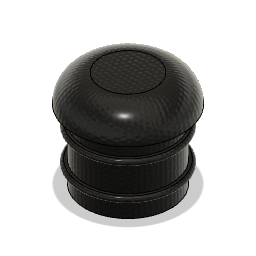
tube_cap (Autodesk Fusion 360 design; units mm, degrees)
Autodesk Fusion 360 part; units mm, degrees
sketch "Esquisse1" plane through (0, 0, 0) normal (0, 1, 0) x (1, 0, 0)
  circle A0 centre (0, 0) radius 8
  circle A1 centre (0, 0) radius 6
  dimension "d1" = 16
  dimension "d2" = 12
  constraint coincident A0.centre A1.centre
  measures "d1" diameter of A0
  measures "d2" diameter of A1
extrude "Extrusion1" add sketch "Esquisse1" along normal blind 10
sketch "Esquisse2" plane through (0, 10, 0) normal (0, 1, 0) x (-1, 0, 0)
  circle A0 centre (0, 0) radius 6
  circle A1 centre (0, 0) radius 8
  circle A2 centre (0, 0) radius 10
  dimension "d5" = 20
  constraint concentric A0 A2
  measures "d5" diameter of A2
extrude "Extrusion2" add sketch "Esquisse2" along normal blind 5 contours A0 | A1 | A2
fillet "Congé1" radius 5 1 edges at (9.3233, 15, -3.6162)
move_face "DécalerLesFaces1" offset -7 1 faces at (7.3035, 0, 0.3974)
sketch "Esquisse3" plane through (0, 7, 0) normal (0, -1, 0) x (1, 0, 0)
  circle A0 centre (0, 0) radius 6
  circle A1 centre (0, 0) radius 8
  circle A2 centre (0, 0) radius 6
  circle A3 centre (0, 0) radius 9
  dimension "d11" = 18
  constraint concentric A0 A2
  constraint coincident A0.centre A1.centre
  measures "d11" diameter of A3
extrude "Extrusion3" add sketch "Esquisse3" along normal blind 1 contours A1 | A3
sketch "Esquisse4" plane through (0, 6, 0) normal (0, -1, 0) x (1, 0, 0)
  circle A0 centre (0, 0) radius 6
  circle A1 centre (0, 0) radius 9
  circle A2 centre (0, 0) radius 6
  circle A3 centre (0, 0) radius 8
  dimension "d14" = 16
  constraint concentric A0 A2
  constraint concentric A0 A3
  measures "d14" diameter of A3
extrude "Extrusion4" add sketch "Esquisse4" along normal blind 5 contours A3
sketch "Esquisse5" plane through (0, 1, 0) normal (0, -1, 0) x (1, 0, 0)
  circle A0 centre (0, 0) radius 6
  circle A1 centre (0, 0) radius 8
  circle A2 centre (0, 0) radius 6
  circle A3 centre (0, 0) radius 9
  constraint concentric A0 A2
  constraint concentric A0 A3
extrude "Extrusion5" add sketch "Esquisse5" along normal blind 1 contours A1 | A3
sketch "Esquisse6" plane through (0, 0, 0) normal (0, -1, 0) x (1, 0, 0)
  circle A0 centre (0, 0) radius 6
  circle A1 centre (0, 0) radius 9
  circle A2 centre (0, 0) radius 6
  circle A3 centre (0, 0) radius 8
  dimension "d19" = 16
  constraint coincident A0.centre A1.centre
  constraint concentric A2 A3
  measures "d19" diameter of A3
extrude "Extrusion6" add sketch "Esquisse6" along normal blind 3 contours A3
fillet "Congé2" radius 0.5 2 edges at (-8.3909, 0, -3.2545) (-8.3909, 6, -3.2545)
fillet "Congé2" radius 0.5 2 edges at (-8.3909, 7, -3.2545) (-8.3909, 1, -3.2545)
